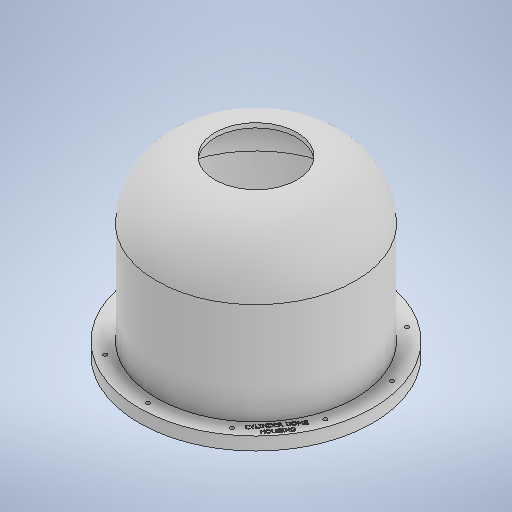
# Autodesk Inventor part: Cylinder Housing
Saved by Autodesk Inventor 2025 (Build 290162000, 162)
## iProperties
Created: 2025-07-09
Part Number: Cylinder Housing
Material: Generic
Document SubType Name: Modeling
Designer: mumin
Density: 1 g/cm^3
Appearance: Default
Author: mumin
Autodesk Inventor part; units mm, degrees
ref_plane "YZ Plane" through (0, 0, 0) normal (1, 0, 0) x (0, 1, 0)
ref_plane "XZ Plane" through (0, 0, 0) normal (0, 1, 0) x (-1, 0, 0)
ref_plane "XY Plane" through (0, 0, 0) normal (0, 0, 1) x (1, 0, 0)
sketch "Sketch1" plane through (0, 0, 0) normal (0, 0, 1) x (1, 0, 0)
  line L0 (110, 0) -> (110, 127.5)
  line L1 (110, 0) -> (135, 0)
  line L2 (135, 0) -> (135, 15)
  line L3 (135, 15) -> (115, 15)
  line L4 (115, 15) -> (115, 132.5)
  line L5 (0, -42.7959) -> (0, 256.7756) projected
  line L6 (0, 200) -> (47.5, 200)
  line L7 (-27, 0) -> (162, 0) projected
  arc A0 (115, 132.5) -> (47.5, 200) centre (47.5, 132.5) ccw
  line L8 (0, 195) -> (42.5, 195)
  arc A1 (110, 127.5) -> (42.5, 195) centre (42.5, 127.5) ccw
  line L9 (0, 200) -> (0, 195)
  point P0 (0, 0)
  dimension "d0" = 135
  dimension "d1" = 110
  dimension "d2" = 115
  dimension "d3" = 15
  dimension "d4" = 200
  dimension "d5" = 67.5
  dimension "d6" = 5
  dimension "d7" = 67.5
  constraints: 16 end point, 4 point on circle, 4 tangent, 3 horizontal, 3 perpendicular, 3 point on line, 2 centre point, 1 collinear, 1 vertical
  measures "d0" distance between parallel lines of L5 L2
  measures "d1" distance between parallel lines of L5 L0
  measures "d2" distance between parallel lines of L5 L4
  measures "d3" distance of L1.end L2.end
  measures "d4" distance between parallel lines of L6 L7
  measures "d5" radius of A0
  measures "d6" distance between parallel lines of L8 L6
  measures "d7" radius of A1
revolve "Revolution1" add sketch "Sketch1" angle 360 about axis through (0, -10, 0) along (0, 1, 0) contours L0 A1 L8 L5 L6 A0 L4 L3 L2 L1
sketch "Sketch2" plane through (0, 200, 0) normal (0, 1, 0) x (1, 0, 0)
  circle A0 centre (0, 0) radius 47.5 projected
extrude "Extrusion1" cut sketch "Sketch2" against normal up to surface
sketch "Sketch3" plane through (0, 15, 0) normal (0, 1, 0) x (1, 0, 0)
  point P0 (0, 0)
  point P1 (0, -125)
  dimension "d11" = 125
  measures "d11" distance of point (0, 0) point (0, -125)
hole "Hole1" at (0, 15, 125) direction (0, -1, 0) diameter 4.5 depth 15
pattern_circular "Circular Pattern1" count 10 over 360 about axis through (0, -10, 0) along (0, 1, 0) of "Hole1"
sketch "Sketch4" plane through (0, 15, 0) normal (0, 1, 0) x (1, 0, 0)
  line L0 (77.8496, -92.0076) -> (110.1579, -49.5047) construction
  line L1 (110.1579, -49.5047) -> (116.6819, -54.4639) construction
  line L2 (116.6819, -54.4639) -> (84.3736, -96.9668) construction
  line L3 (84.3736, -96.9668) -> (77.8496, -92.0076) construction
  spline S0 degree 2 poles (83.8059, -92.7556) (83.5117, -93.1427) (82.7526, -93.5989) (82.3099, -93.639) knots 0 0 0 1 2 2 2
  spline S1 degree 2 poles (82.3099, -93.639) (81.8704, -93.6815) (80.8976, -93.3543) (80.3944, -92.9718) knots 0 0 0 1 2 2 2
  spline S2 degree 2 poles (80.3944, -92.9718) (79.8944, -92.5917) (79.3462, -91.7729) (79.2559, -91.3226) knots 0 0 0 1 2 2 2
  spline S3 degree 2 poles (79.2559, -91.3226) (79.1696, -90.8804) (79.3843, -90.0154) (79.6908, -89.6122) knots 0 0 0 1 2 2 2
  spline S4 degree 2 poles (79.6908, -89.6122) (79.8428, -89.4122) (80.1681, -89.1048) (80.3261, -88.9907) knots 0 0 0 1 2 2 2
  spline S5 degree 2 poles (80.3261, -88.9907) (80.4661, -88.8936) (80.789, -88.7166) (80.9605, -88.6382) knots 0 0 0 1 2 2 2
  line L4 (80.9605, -88.6382) -> (81.5992, -89.1237)
  line L5 (81.5992, -89.1237) -> (81.5673, -89.1657)
  spline S6 degree 2 poles (81.5673, -89.1657) (81.4488, -89.1876) (81.1014, -89.2696) (80.8942, -89.3615) knots 0 0 0 1 2 2 2
  spline S7 degree 2 poles (80.8942, -89.3615) (80.6951, -89.4493) (80.3165, -89.7265) (80.1399, -89.9587) knots 0 0 0 1 2 2 2
  spline S8 degree 2 poles (80.1399, -89.9587) (79.9462, -90.2136) (79.8102, -90.8278) (79.8802, -91.1508) knots 0 0 0 1 2 2 2
  spline S9 degree 2 poles (79.8802, -91.1508) (79.9559, -91.473) (80.4298, -92.1284) (80.8137, -92.4202) knots 0 0 0 1 2 2 2
  spline S10 degree 2 poles (80.8137, -92.4202) (81.2233, -92.7316) (81.9632, -92.9835) (82.2964, -92.9671) knots 0 0 0 1 2 2 2
  spline S11 degree 2 poles (82.2964, -92.9671) (82.6207, -92.9489) (83.1615, -92.6525) (83.3527, -92.4009) knots 0 0 0 1 2 2 2
  spline S12 degree 2 poles (83.3527, -92.4009) (83.5268, -92.1719) (83.7106, -91.6958) (83.742, -91.4804) knots 0 0 0 1 2 2 2
  spline S13 degree 2 poles (83.742, -91.4804) (83.7685, -91.2715) (83.7586, -90.923) (83.7439, -90.8151) knots 0 0 0 1 2 2 2
  line L6 (83.7439, -90.8151) -> (83.7733, -90.7764)
  line L7 (83.7733, -90.7764) -> (84.4055, -91.257)
  spline S14 degree 2 poles (84.4055, -91.257) (84.3663, -91.4358) (84.3026, -91.7539) (84.2292, -91.9576) knots 0 0 0 1 2 2 2
  spline S15 degree 2 poles (84.2292, -91.9576) (84.1549, -92.176) (83.9873, -92.5169) (83.8059, -92.7556) knots 0 0 0 1 2 2 2
  line L8 (83.1896, -85.1566) -> (84.3865, -88.1887)
  line L9 (84.3865, -88.1887) -> (86.1477, -89.5275)
  line L10 (86.1477, -89.5275) -> (85.7456, -90.0565)
  line L11 (85.7456, -90.0565) -> (84.0392, -88.7594)
  line L12 (84.0392, -88.7594) -> (80.7425, -88.3759)
  line L13 (80.7425, -88.3759) -> (81.1888, -87.7888)
  line L14 (81.1888, -87.7888) -> (83.7226, -88.0912)
  line L15 (83.7226, -88.0912) -> (82.763, -85.7179)
  line L16 (82.763, -85.7179) -> (83.1896, -85.1566)
  line L17 (89.2029, -85.5083) -> (87.4497, -87.8147)
  line L18 (87.4497, -87.8147) -> (83.4692, -84.7889)
  line L19 (83.4692, -84.7889) -> (83.8713, -84.2599)
  line L20 (83.8713, -84.2599) -> (87.3809, -86.9277)
  line L21 (87.3809, -86.9277) -> (88.7319, -85.1503)
  line L22 (88.7319, -85.1503) -> (89.2029, -85.5083)
  line L23 (90.5736, -83.7051) -> (89.4015, -85.247)
  line L24 (89.4015, -85.247) -> (88.9951, -84.938)
  line L25 (88.9951, -84.938) -> (89.38, -84.4316)
  line L26 (89.38, -84.4316) -> (86.2124, -82.0237)
  line L27 (86.2124, -82.0237) -> (85.8274, -82.5302)
  line L28 (85.8274, -82.5302) -> (85.421, -82.2212)
  line L29 (85.421, -82.2212) -> (86.593, -80.6793)
  line L30 (86.593, -80.6793) -> (86.9995, -80.9883)
  line L31 (86.9995, -80.9883) -> (86.6145, -81.4947)
  line L32 (86.6145, -81.4947) -> (89.7822, -83.9026)
  line L33 (89.7822, -83.9026) -> (90.1671, -83.3961)
  line L34 (90.1671, -83.3961) -> (90.5736, -83.7051)
  line L35 (93.2364, -80.202) -> (92.7853, -80.7955)
  line L36 (92.7853, -80.7955) -> (88.0143, -79.9478)
  line L37 (88.0143, -79.9478) -> (91.4465, -82.5567)
  line L38 (91.4465, -82.5567) -> (91.0713, -83.0503)
  line L39 (91.0713, -83.0503) -> (87.0908, -80.0245)
  line L40 (87.0908, -80.0245) -> (87.6621, -79.2729)
  line L41 (87.6621, -79.2729) -> (92.0323, -80.0653)
  line L42 (92.0323, -80.0653) -> (88.8808, -77.6697)
  line L43 (88.8808, -77.6697) -> (89.2559, -77.1762)
  line L44 (89.2559, -77.1762) -> (93.2364, -80.202)
  spline S16 degree 2 poles (94.2482, -74.7465) (94.7934, -75.1609) (95.3348, -76.2697) (95.298, -76.827) knots 0 0 0 1 2 2 2
  spline S17 degree 2 poles (95.298, -76.827) (95.2578, -77.2749) (94.9136, -77.9956) (94.5458, -78.4794) knots 0 0 0 1 2 2 2
  line L45 (94.5458, -78.4794) -> (93.8494, -79.3955)
  line L46 (93.8494, -79.3955) -> (89.8689, -76.3698)
  line L47 (89.8689, -76.3698) -> (90.5579, -75.4633)
  spline S18 degree 2 poles (90.5579, -75.4633) (90.9846, -74.9021) (91.6378, -74.3909) (91.9578, -74.2779) knots 0 0 0 1 2 2 2
  spline S19 degree 2 poles (91.9578, -74.2779) (92.5045, -74.0877) (93.6676, -74.3051) (94.2482, -74.7465) knots 0 0 0 1 2 2 2
  spline S20 degree 2 poles (93.8225, -75.2932) (93.3644, -74.945) (92.4856, -74.7553) (92.0737, -74.9156) knots 0 0 0 1 2 2 2
  spline S21 degree 2 poles (92.0737, -74.9156) (91.786, -75.0328) (91.3078, -75.4277) (91.0356, -75.7857) knots 0 0 0 1 2 2 2
  line L48 (91.0356, -75.7857) -> (90.7291, -76.1889)
  line L49 (90.7291, -76.1889) -> (93.7935, -78.5183)
  line L50 (93.7935, -78.5183) -> (94.1, -78.1151)
  spline S22 degree 2 poles (94.1, -78.1151) (94.3673, -77.7635) (94.659, -77.1454) (94.6717, -76.8141) knots 0 0 0 1 2 2 2
  spline S23 degree 2 poles (94.6717, -76.8141) (94.6954, -76.3945) (94.287, -75.6463) (93.8225, -75.2932) knots 0 0 0 1 2 2 2
  line L51 (96.6717, -75.6827) -> (92.6912, -72.657)
  line L52 (92.6912, -72.657) -> (94.5841, -70.1667)
  line L53 (94.5841, -70.1667) -> (95.0551, -70.5247)
  line L54 (95.0551, -70.5247) -> (93.5643, -72.4859)
  line L55 (93.5643, -72.4859) -> (94.6545, -73.3147)
  line L56 (94.6545, -73.3147) -> (96.0448, -71.4857)
  line L57 (96.0448, -71.4857) -> (96.5158, -71.8437)
  line L58 (96.5158, -71.8437) -> (95.1255, -73.6727)
  line L59 (95.1255, -73.6727) -> (96.6029, -74.7957)
  line L60 (96.6029, -74.7957) -> (98.0937, -72.8345)
  line L61 (98.0937, -72.8345) -> (98.5647, -73.1925)
  line L62 (98.5647, -73.1925) -> (96.6717, -75.6827)
  line L63 (101.3477, -69.5313) -> (100.8254, -70.2184)
  line L64 (100.8254, -70.2184) -> (98.2853, -70.2725)
  line L65 (98.2853, -70.2725) -> (97.8243, -70.8789)
  line L66 (97.8243, -70.8789) -> (99.4081, -72.0828)
  line L67 (99.4081, -72.0828) -> (99.006, -72.6118)
  line L68 (99.006, -72.6118) -> (95.0255, -69.5861)
  line L69 (95.0255, -69.5861) -> (95.8052, -68.5603)
  spline S24 degree 2 poles (95.8052, -68.5603) (96.0651, -68.2184) (96.49, -67.8135) (96.7848, -67.7068) knots 0 0 0 1 2 2 2
  spline S25 degree 2 poles (96.7848, -67.7068) (97.0797, -67.6001) (97.6861, -67.6794) (97.999, -67.9172) knots 0 0 0 1 2 2 2
  spline S26 degree 2 poles (97.999, -67.9172) (98.4345, -68.2483) (98.6864, -69.1421) (98.539, -69.6306) knots 0 0 0 1 2 2 2
  line L70 (98.539, -69.6306) -> (101.3477, -69.5313)
  spline S27 degree 2 poles (97.6217, -68.5007) (97.4475, -68.3683) (97.0866, -68.2874) (96.9014, -68.3502) knots 0 0 0 1 2 2 2
  spline S28 degree 2 poles (96.9014, -68.3502) (96.7414, -68.4067) (96.4521, -68.6601) (96.2853, -68.8794) knots 0 0 0 1 2 2 2
  line L71 (96.2853, -68.8794) -> (95.8857, -69.4052)
  line L72 (95.8857, -69.4052) -> (97.3824, -70.543)
  line L73 (97.3824, -70.543) -> (97.7355, -70.0785)
  spline S29 degree 2 poles (97.7355, -70.0785) (97.9096, -69.8494) (98.106, -69.4236) (98.0758, -69.2022) knots 0 0 0 1 2 2 2
  spline S30 degree 2 poles (98.0758, -69.2022) (98.0544, -69.0027) (97.8281, -68.6576) (97.6217, -68.5007) knots 0 0 0 1 2 2 2
  spline S31 degree 2 poles (103.2863, -62.8565) (103.8314, -63.2709) (104.3729, -64.3797) (104.3361, -64.937) knots 0 0 0 1 2 2 2
  spline S32 degree 2 poles (104.3361, -64.937) (104.2959, -65.3849) (103.9517, -66.1056) (103.5839, -66.5894) knots 0 0 0 1 2 2 2
  line L74 (103.5839, -66.5894) -> (102.8875, -67.5055)
  line L75 (102.8875, -67.5055) -> (98.907, -64.4798)
  line L76 (98.907, -64.4798) -> (99.596, -63.5733)
  spline S33 degree 2 poles (99.596, -63.5733) (100.0227, -63.0121) (100.6759, -62.5009) (100.9959, -62.3879) knots 0 0 0 1 2 2 2
  spline S34 degree 2 poles (100.9959, -62.3879) (101.5425, -62.1977) (102.7057, -62.4151) (103.2863, -62.8565) knots 0 0 0 1 2 2 2
  spline S35 degree 2 poles (102.8606, -63.4032) (102.4025, -63.055) (101.5236, -62.8653) (101.1117, -63.0256) knots 0 0 0 1 2 2 2
  spline S36 degree 2 poles (101.1117, -63.0256) (100.8241, -63.1428) (100.3459, -63.5377) (100.0737, -63.8957) knots 0 0 0 1 2 2 2
  line L77 (100.0737, -63.8957) -> (99.7672, -64.2989)
  line L78 (99.7672, -64.2989) -> (102.8316, -66.6283)
  line L79 (102.8316, -66.6283) -> (103.1381, -66.2251)
  spline S37 degree 2 poles (103.1381, -66.2251) (103.4054, -65.8735) (103.6971, -65.2554) (103.7097, -64.9241) knots 0 0 0 1 2 2 2
  spline S38 degree 2 poles (103.7097, -64.9241) (103.7335, -64.5044) (103.3251, -63.7563) (102.8606, -63.4032) knots 0 0 0 1 2 2 2
  spline S39 degree 2 poles (104.3247, -58.2966) (104.7608, -58.2719) (105.7263, -58.6088) (106.223, -58.9864) knots 0 0 0 1 2 2 2
  spline S40 degree 2 poles (106.223, -58.9864) (106.7069, -59.3542) (107.3044, -60.1952) (107.3924, -60.6285) knots 0 0 0 1 2 2 2
  spline S41 degree 2 poles (107.3924, -60.6285) (107.4834, -61.0845) (107.2551, -61.934) (106.9584, -62.3243) knots 0 0 0 1 2 2 2
  spline S42 degree 2 poles (106.9584, -62.3243) (106.6519, -62.7275) (105.8873, -63.1642) (105.4406, -63.1962) knots 0 0 0 1 2 2 2
  spline S43 degree 2 poles (105.4406, -63.1962) (105.002, -63.2241) (104.0382, -62.8783) (103.5479, -62.5056) knots 0 0 0 1 2 2 2
  spline S44 degree 2 poles (103.5479, -62.5056) (103.0479, -62.1256) (102.4754, -61.2985) (102.3753, -60.8611) knots 0 0 0 1 2 2 2
  spline S45 degree 2 poles (102.3753, -60.8611) (102.2874, -60.4278) (102.506, -59.571) (102.8101, -59.171) knots 0 0 0 1 2 2 2
  spline S46 degree 2 poles (102.8101, -59.171) (103.1191, -58.7645) (103.8982, -58.3287) (104.3247, -58.2966) knots 0 0 0 1 2 2 2
  spline S47 degree 2 poles (105.8037, -59.538) (105.4102, -59.2388) (104.6706, -58.9464) (104.3529, -58.9492) knots 0 0 0 1 2 2 2
  spline S48 degree 2 poles (104.3529, -58.9492) (104.0263, -58.9503) (103.4815, -59.2385) (103.2706, -59.5159) knots 0 0 0 1 2 2 2
  spline S49 degree 2 poles (103.2706, -59.5159) (103.0524, -59.803) (102.9238, -60.3873) (103.0116, -60.7136) knots 0 0 0 1 2 2 2
  spline S50 degree 2 poles (103.0116, -60.7136) (103.0947, -61.0262) (103.5801, -61.6598) (103.9672, -61.954) knots 0 0 0 1 2 2 2
  spline S51 degree 2 poles (103.9672, -61.954) (104.751, -62.5499) (106.0835, -62.5245) (106.5028, -61.9729) knots 0 0 0 1 2 2 2
  spline S52 degree 2 poles (106.5028, -61.9729) (106.9221, -61.4213) (106.5876, -60.1338) (105.8037, -59.538) knots 0 0 0 1 2 2 2
  line L80 (111.2489, -56.5058) -> (110.8468, -57.0348)
  line L81 (110.8468, -57.0348) -> (107.4178, -54.4284)
  line L82 (107.4178, -54.4284) -> (108.9605, -57.2398)
  line L83 (108.9605, -57.2398) -> (108.7153, -57.5624)
  line L84 (108.7153, -57.5624) -> (105.6009, -56.8186)
  line L85 (105.6009, -56.8186) -> (109.0298, -59.4251)
  line L86 (109.0298, -59.4251) -> (108.6547, -59.9186)
  line L87 (108.6547, -59.9186) -> (104.6741, -56.8929)
  line L88 (104.6741, -56.8929) -> (105.2234, -56.1703)
  line L89 (105.2234, -56.1703) -> (108.1947, -56.8613)
  line L90 (108.1947, -56.8613) -> (106.7093, -54.2155)
  line L91 (106.7093, -54.2155) -> (107.2683, -53.4801)
  line L92 (107.2683, -53.4801) -> (111.2489, -56.5058)
  line L93 (111.8619, -55.6994) -> (107.8813, -52.6736)
  line L94 (107.8813, -52.6736) -> (109.7743, -50.1834)
  line L95 (109.7743, -50.1834) -> (110.2452, -50.5414)
  line L96 (110.2452, -50.5414) -> (108.7544, -52.5026)
  line L97 (108.7544, -52.5026) -> (109.8447, -53.3314)
  line L98 (109.8447, -53.3314) -> (111.235, -51.5024)
  line L99 (111.235, -51.5024) -> (111.706, -51.8604)
  line L100 (111.706, -51.8604) -> (110.3157, -53.6894)
  line L101 (110.3157, -53.6894) -> (111.7931, -54.8124)
  line L102 (111.7931, -54.8124) -> (113.2839, -52.8511)
  line L103 (113.2839, -52.8511) -> (113.7548, -53.2091)
  line L104 (113.7548, -53.2091) -> (111.8619, -55.6994)
  line L105 (98.1707, -87.3144) -> (97.7686, -87.8434)
  line L106 (97.7686, -87.8434) -> (95.8203, -86.3624)
  line L107 (95.8203, -86.3624) -> (94.4275, -88.1946)
  line L108 (94.4275, -88.1946) -> (96.3759, -89.6756)
  line L109 (96.3759, -89.6756) -> (95.9738, -90.2047)
  line L110 (95.9738, -90.2047) -> (91.9932, -87.1789)
  line L111 (91.9932, -87.1789) -> (92.3953, -86.6499)
  line L112 (92.3953, -86.6499) -> (93.9566, -87.8366)
  line L113 (93.9566, -87.8366) -> (95.3493, -86.0044)
  line L114 (95.3493, -86.0044) -> (93.7881, -84.8177)
  line L115 (93.7881, -84.8177) -> (94.1902, -84.2886)
  line L116 (94.1902, -84.2886) -> (98.1707, -87.3144)
  spline S53 degree 2 poles (97.3986, -81.0119) (97.8348, -80.9872) (98.8002, -81.324) (99.297, -81.7016) knots 0 0 0 1 2 2 2
  spline S54 degree 2 poles (99.297, -81.7016) (99.7808, -82.0694) (100.3783, -82.9104) (100.4663, -83.3437) knots 0 0 0 1 2 2 2
  spline S55 degree 2 poles (100.4663, -83.3437) (100.5574, -83.7998) (100.329, -84.6492) (100.0323, -85.0395) knots 0 0 0 1 2 2 2
  spline S56 degree 2 poles (100.0323, -85.0395) (99.7258, -85.4427) (98.9612, -85.8795) (98.5145, -85.9114) knots 0 0 0 1 2 2 2
  spline S57 degree 2 poles (98.5145, -85.9114) (98.0759, -85.9394) (97.1121, -85.5936) (96.6218, -85.2209) knots 0 0 0 1 2 2 2
  spline S58 degree 2 poles (96.6218, -85.2209) (96.1219, -84.8408) (95.5494, -84.0138) (95.4493, -83.5763) knots 0 0 0 1 2 2 2
  spline S59 degree 2 poles (95.4493, -83.5763) (95.3613, -83.143) (95.58, -82.2862) (95.884, -81.8862) knots 0 0 0 1 2 2 2
  spline S60 degree 2 poles (95.884, -81.8862) (96.193, -81.4798) (96.9722, -81.044) (97.3986, -81.0119) knots 0 0 0 1 2 2 2
  spline S61 degree 2 poles (98.8777, -82.2532) (98.4841, -81.9541) (97.7445, -81.6616) (97.4268, -81.6644) knots 0 0 0 1 2 2 2
  spline S62 degree 2 poles (97.4268, -81.6644) (97.1002, -81.6656) (96.5554, -81.9538) (96.3446, -82.2312) knots 0 0 0 1 2 2 2
  spline S63 degree 2 poles (96.3446, -82.2312) (96.1263, -82.5183) (95.9977, -83.1026) (96.0856, -83.4289) knots 0 0 0 1 2 2 2
  spline S64 degree 2 poles (96.0856, -83.4289) (96.1687, -83.7414) (96.654, -84.3751) (97.0411, -84.6693) knots 0 0 0 1 2 2 2
  spline S65 degree 2 poles (97.0411, -84.6693) (97.825, -85.2651) (99.1574, -85.2397) (99.5767, -84.6881) knots 0 0 0 1 2 2 2
  spline S66 degree 2 poles (99.5767, -84.6881) (99.996, -84.1365) (99.6615, -82.8491) (98.8777, -82.2532) knots 0 0 0 1 2 2 2
  spline S67 degree 2 poles (102.8693, -81.3074) (102.602, -81.659) (102.0209, -82.0418) (101.6973, -82.0859) knots 0 0 0 1 2 2 2
  spline S68 degree 2 poles (101.6973, -82.0859) (101.3315, -82.1386) (100.6209, -81.8682) (100.1951, -81.5445) knots 0 0 0 1 2 2 2
  line L117 (100.1951, -81.5445) -> (97.7113, -79.6565)
  line L118 (97.7113, -79.6565) -> (98.1134, -79.1275)
  line L119 (98.1134, -79.1275) -> (100.5972, -81.0155)
  spline S69 degree 2 poles (100.5972, -81.0155) (100.8746, -81.2264) (101.3028, -81.4399) (101.5304, -81.4551) knots 0 0 0 1 2 2 2
  spline S70 degree 2 poles (101.5304, -81.4551) (101.7726, -81.4713) (102.2166, -81.2286) (102.4177, -80.9641) knots 0 0 0 1 2 2 2
  spline S71 degree 2 poles (102.4177, -80.9641) (102.6065, -80.7157) (102.7362, -80.2036) (102.6559, -79.9745) knots 0 0 0 1 2 2 2
  spline S72 degree 2 poles (102.6559, -79.9745) (102.5803, -79.7593) (102.2632, -79.4063) (101.9955, -79.2028) knots 0 0 0 1 2 2 2
  line L120 (101.9955, -79.2028) -> (99.4988, -77.305)
  line L121 (99.4988, -77.305) -> (99.9009, -76.7759)
  line L122 (99.9009, -76.7759) -> (102.3847, -78.664)
  spline S73 degree 2 poles (102.3847, -78.664) (102.8009, -78.9803) (103.2669, -79.5992) (103.3083, -79.9666) knots 0 0 0 1 2 2 2
  spline S74 degree 2 poles (103.3083, -79.9666) (103.3507, -80.2991) (103.1488, -80.9396) (102.8693, -81.3074) knots 0 0 0 1 2 2 2
  spline S75 degree 2 poles (105.3721, -77.988) (105.0436, -78.4202) (104.402, -78.8893) (104.0694, -79.059) knots 0 0 0 1 2 2 2
  line L123 (104.0694, -79.059) -> (103.4049, -78.5539)
  line L124 (103.4049, -78.5539) -> (103.4343, -78.5152)
  spline S76 degree 2 poles (103.4343, -78.5152) (103.8781, -78.4402) (104.6517, -77.9849) (104.8847, -77.6785) knots 0 0 0 1 2 2 2
  spline S77 degree 2 poles (104.8847, -77.6785) (105.2181, -77.2398) (105.1945, -76.5143) (104.8945, -76.2863) knots 0 0 0 1 2 2 2
  spline S78 degree 2 poles (104.8945, -76.2863) (104.6558, -76.1049) (104.18, -76.1147) (103.9121, -76.3132) knots 0 0 0 1 2 2 2
  spline S79 degree 2 poles (103.9121, -76.3132) (103.7207, -76.4578) (103.4168, -76.7103) (103.1847, -76.8952) knots 0 0 0 1 2 2 2
  spline S80 degree 2 poles (103.1847, -76.8952) (102.9729, -77.06) (102.5607, -77.2607) (102.3329, -77.286) knots 0 0 0 1 2 2 2
  spline S81 degree 2 poles (102.3329, -77.286) (102.1074, -77.308) (101.6496, -77.1738) (101.4174, -76.9972) knots 0 0 0 1 2 2 2
  spline S82 degree 2 poles (101.4174, -76.9972) (100.9335, -76.6294) (100.8525, -75.3769) (101.2963, -74.793) knots 0 0 0 1 2 2 2
  spline S83 degree 2 poles (101.2963, -74.793) (101.5513, -74.4575) (102.1347, -73.9645) (102.4542, -73.8053) knots 0 0 0 1 2 2 2
  line L125 (102.4542, -73.8053) -> (103.0865, -74.2859)
  line L126 (103.0865, -74.2859) -> (103.057, -74.3246)
  spline S84 degree 2 poles (103.057, -74.3246) (102.7382, -74.3825) (102.0289, -74.7799) (101.7813, -75.1057) knots 0 0 0 1 2 2 2
  spline S85 degree 2 poles (101.7813, -75.1057) (101.5018, -75.4734) (101.5012, -76.1906) (101.7818, -76.404) knots 0 0 0 1 2 2 2
  spline S86 degree 2 poles (101.7818, -76.404) (102.0334, -76.5952) (102.5369, -76.5555) (102.7959, -76.3554) knots 0 0 0 1 2 2 2
  spline S87 degree 2 poles (102.7959, -76.3554) (102.9686, -76.222) (103.455, -75.8232) (103.626, -75.6987) knots 0 0 0 1 2 2 2
  spline S88 degree 2 poles (103.626, -75.6987) (104.0632, -75.3846) (104.8589, -75.389) (105.2299, -75.671) knots 0 0 0 1 2 2 2
  spline S89 degree 2 poles (105.2299, -75.671) (105.4654, -75.8499) (105.7723, -76.3835) (105.8004, -76.6747) knots 0 0 0 1 2 2 2
  spline S90 degree 2 poles (105.8004, -76.6747) (105.8299, -76.9974) (105.6492, -77.6235) (105.3721, -77.988) knots 0 0 0 1 2 2 2
  line L127 (107.8292, -74.6083) -> (106.6571, -76.1502)
  line L128 (106.6571, -76.1502) -> (106.2507, -75.8412)
  line L129 (106.2507, -75.8412) -> (106.6357, -75.3348)
  line L130 (106.6357, -75.3348) -> (103.468, -72.9269)
  line L131 (103.468, -72.9269) -> (103.083, -73.4334)
  line L132 (103.083, -73.4334) -> (102.6766, -73.1244)
  line L133 (102.6766, -73.1244) -> (103.8487, -71.5825)
  line L134 (103.8487, -71.5825) -> (104.2551, -71.8915)
  line L135 (104.2551, -71.8915) -> (103.8701, -72.3979)
  line L136 (103.8701, -72.3979) -> (107.0378, -74.8058)
  line L137 (107.0378, -74.8058) -> (107.4228, -74.2993)
  line L138 (107.4228, -74.2993) -> (107.8292, -74.6083)
  line L139 (110.4921, -71.1052) -> (110.0409, -71.6987)
  line L140 (110.0409, -71.6987) -> (105.2699, -70.851)
  line L141 (105.2699, -70.851) -> (108.7021, -73.4599)
  line L142 (108.7021, -73.4599) -> (108.327, -73.9535)
  line L143 (108.327, -73.9535) -> (104.3464, -70.9277)
  line L144 (104.3464, -70.9277) -> (104.9177, -70.1761)
  line L145 (104.9177, -70.1761) -> (109.2879, -70.9685)
  line L146 (109.2879, -70.9685) -> (106.1364, -68.5729)
  line L147 (106.1364, -68.5729) -> (106.5115, -68.0794)
  line L148 (106.5115, -68.0794) -> (110.4921, -71.1052)
  spline S91 degree 2 poles (112.4502, -68.6899) (112.129, -69.1125) (111.3388, -69.6163) (110.8863, -69.6693) knots 0 0 0 1 2 2 2
  spline S92 degree 2 poles (110.8863, -69.6693) (110.4305, -69.7198) (109.4464, -69.3942) (108.9399, -69.0092) knots 0 0 0 1 2 2 2
  spline S93 degree 2 poles (108.9399, -69.0092) (108.4593, -68.6439) (107.904, -67.7942) (107.8243, -67.3366) knots 0 0 0 1 2 2 2
  spline S94 degree 2 poles (107.8243, -67.3366) (107.7469, -66.8961) (108.0025, -65.9707) (108.3237, -65.5481) knots 0 0 0 1 2 2 2
  spline S95 degree 2 poles (108.3237, -65.5481) (108.4782, -65.3449) (108.8158, -65.0213) (108.9949, -64.8928) knots 0 0 0 1 2 2 2
  spline S96 degree 2 poles (108.9949, -64.8928) (109.1366, -64.7867) (109.5286, -64.5656) (109.6563, -64.5048) knots 0 0 0 1 2 2 2
  line L149 (109.6563, -64.5048) -> (110.2949, -64.9903)
  line L150 (110.2949, -64.9903) -> (110.2606, -65.0355)
  spline S97 degree 2 poles (110.2606, -65.0355) (110.0975, -65.0693) (109.7801, -65.1588) (109.5426, -65.2837) knots 0 0 0 1 2 2 2
  spline S98 degree 2 poles (109.5426, -65.2837) (109.3394, -65.3837) (108.9166, -65.7189) (108.7352, -65.9576) knots 0 0 0 1 2 2 2
  spline S99 degree 2 poles (108.7352, -65.9576) (108.2987, -66.5317) (108.6238, -67.8985) (109.3431, -68.4453) knots 0 0 0 1 2 2 2
  spline S100 degree 2 poles (109.3431, -68.4453) (109.7431, -68.7494) (110.4853, -69.0184) (110.8266, -68.9979) knots 0 0 0 1 2 2 2
  spline S101 degree 2 poles (110.8266, -68.9979) (111.163, -68.9839) (111.7469, -68.6643) (111.9774, -68.3611) knots 0 0 0 1 2 2 2
  spline S102 degree 2 poles (111.9774, -68.3611) (112.1466, -68.1385) (112.4205, -67.6443) (112.4712, -67.4436) knots 0 0 0 1 2 2 2
  line L151 (112.4712, -67.4436) -> (111.4422, -66.6615)
  line L152 (111.4422, -66.6615) -> (110.7409, -67.584)
  line L153 (110.7409, -67.584) -> (110.2764, -67.2309)
  line L154 (110.2764, -67.2309) -> (111.3749, -65.7858)
  line L155 (111.3749, -65.7858) -> (113.1136, -67.1074)
  spline S103 degree 2 poles (113.1136, -67.1074) (113.0827, -67.2418) (112.9615, -67.6891) (112.8931, -67.8662) knots 0 0 0 1 2 2 2
  spline S104 degree 2 poles (112.8931, -67.8662) (112.8016, -68.1071) (112.6194, -68.4673) (112.4502, -68.6899) knots 0 0 0 1 2 2 2
  point P0 (0, 0)
  constraints: 2 other
emboss "Emboss1" sketch "Sketch4" operation cut depth 1 direction (0, -1, 0)
body "Solid1"
